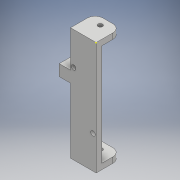
# Autodesk Inventor part: mtv_axelHolder(pushingAxel)1-13
Saved by Autodesk Inventor 2018 (Build 220112000, 112)
## iProperties
Created: 2019-01-14
Part Number: mtv_axelHolder(pushingAxel)1-13
Material: Generic
Document SubType Name: Modeling
Designer: aditya
Density: 1 g/cm^3
Appearance: Default
Author: aditya
## iProperties of the stored document mtv_axelHolder(pushingAxel)1-13_3DPrint.ipt
Created: 2019-01-14
Part Number: mtv_axelHolder(pushingAxel)1-13_3DPrint
Material: Generic
Document SubType Name: Modeling
Designer: aditya
Density: 1 g/cm^3
Appearance: Default
Author: aditya
Autodesk Inventor part; units mm, degrees
ref_plane "YZ Plane" through (0, 0, 0) normal (1, 0, 0) x (0, 1, 0)
ref_plane "XZ Plane" through (0, 0, 0) normal (0, 1, 0) x (-1, 0, 0)
ref_plane "XY Plane" through (0, 0, 0) normal (0, 0, 1) x (1, 0, 0)
sketch "Sketch1" plane through (0, 0, 0) normal (0, 1, 0) x (-1, 0, 0)
  line L0 (0, 0) -> (22.65, 0)
  line L1 (22.65, 0) -> (22.65, -100)
  line L2 (22.65, -100) -> (0, -100)
  line L3 (0, -100) -> (0, 0)
  dimension "d0" = 22.65
  dimension "d1" = 100
  constraints: 8 end point, 2 parallel, 1 horizontal, 1 perpendicular
  measures "d0" distance of L1.end L2.end
  measures "d1" distance of L0.end L1.end
extrude "Extrusion1" add sketch "Sketch1" along normal blind 5
sketch "Sketch2" plane through (0, 5, 0) normal (0, 1, 0) x (1, 0, 0)
  line L0 (-22.65, 0) -> (0, 0) projected
  line L1 (0, 0) -> (0, 100) projected
  line L2 (-22.65, 0) -> (0, 0)
  line L3 (0, 0) -> (0, 5)
  line L4 (0, 5) -> (-22.65, 5)
  line L5 (-22.65, 5) -> (-22.65, 0)
  line L6 (-22.65, 100) -> (-22.65, 0) projected
  line L7 (-22.65, 100) -> (0, 100)
  line L8 (0, 100) -> (0, 95)
  line L9 (0, 95) -> (-22.65, 95)
  line L10 (-22.65, 95) -> (-22.65, 100)
  dimension "d4" = 5
  dimension "d5" = 5
  constraints: 16 end point, 4 parallel, 2 horizontal, 2 perpendicular, 2 point on line
  measures "d4" distance of L3.end L2.end
  measures "d5" distance of L7.end L8.end
extrude "Extrusion2" add sketch "Sketch2" along normal blind 40 contours L5 L4 L1 L0 | L6 L7 L1 L9
sketch "Sketch3" plane through (-22.65, 0, 0) normal (0, 0, 1) x (1, 0, 0)
  point P0 (22.65, 0)
sketch "Sketch4" plane through (-22.65, 0, 0) normal (0, 0, 1) x (1, 0, 0)
  line L0 (22.65, 0) -> (0, 0) projected
  line L1 (22.65, 0) -> (0, 0)
  line L2 (0, 0) -> (11.325, 0)
  line L3 (11.325, 0) -> (11.325, 45)
  line L4 (22.65, 45) -> (0, 45) projected
  line L5 (0, 5) -> (22.65, 5) projected
  line L6 (22.65, 5) -> (0, 5)
  line L7 (11.325, 5) -> (11.325, 15) construction
  dimension "d8" = 10
  constraints: 10 end point, 3 midpoint, 1 collinear, 1 horizontal, 1 point on line
  measures "d8" distance of L7.start L7.end
hole "Hole1" at (-11.325, 15, 0) direction (0, 0, -1) diameter 4 depth 115 tip angle 118
sketch "Sketch5" plane through (-22.65, 0, 0) normal (0, 0, 1) x (1, 0, 0)
  line L0 (0, 5) -> (0, 45) projected
  line L1 (0, 45) -> (23, 45)
  line L2 (23, 45) -> (23, 21.7538)
  line L3 (23, 21.7538) -> (0, 21.7538)
  line L4 (0, 21.7538) -> (0, 45)
  point P0 (22.65, 0)
  dimension "d16" = 23
  constraints: 8 end point, 2 parallel, 1 horizontal, 1 perpendicular
  measures "d16" distance of L2.end L3.end
extrude "Extrusion3" cut sketch "Sketch5" against normal blind 102.75
sketch "Sketch6" plane through (0, 5, 0) normal (0, 1, 0) x (1, 0, 0)
  line L0 (0, 95) -> (-22.65, 95) construction
  line L1 (-22.65, 5) -> (0, 5) construction
  line L2 (0, 95) -> (0, 5) construction
  line L3 (0, 5) -> (-1.175, 5) construction
  line L4 (-1.175, 5) -> (-1.175, 95) construction
  line L5 (-1.175, 50) -> (-22.65, 50) construction
  line L6 (-22.65, 95) -> (-22.65, 5) construction
  line L7 (0, 5) -> (0, 95) construction
  line L8 (0, 5) -> (-22.65, 5) construction
  line L9 (-13.325, 5) -> (-9.325, 5) construction
  line L10 (-11.325, 5) -> (-11.325, 95) construction
  line L11 (-11.325, 50) -> (-2.825, 50) construction
  line L12 (-2.825, 50) -> (-2.825, 71) construction
  line L13 (-11.325, 50) -> (-19.825, 50) construction
  line L14 (-11.325, 50) -> (-2.825, 50) construction
  line L15 (-19.825, 50) -> (-19.825, 29) construction
  point P0 (0, 0)
  dimension "d19" = 1.175
  dimension "d20" = 8.5
  dimension "d21" = 21
  dimension "d22" = 90
  dimension "d23" = 8.5
  dimension "d24" = 180
  dimension "d25" = 21
  constraints: 22 end point, 5 midpoint, 3 coincident, 2 collinear, 2 parallel, 2 perpendicular, 2 point on line, 1 horizontal, 1 vertical
  measures "d19" distance of L1.end L3.end
  measures "d20" distance of L11.start L11.end
  measures "d21" distance of L11.end L12.end
  measures "d22" angle of L12 L11
  measures "d23" distance of L11.start L13.end
  measures "d24" angle of L13 L14
  measures "d25" distance of L13.end L15.end
hole "Hole2" at (-2.825, 5, -71) at (-19.825, 5, -29) direction (0, -1, 0) diameter 4 depth 115 tip angle 118
fillet "Fillet1" radius 1 2 edges at (-2.825, 5, -73) (-19.825, 5, -31)
sketch "Sketch7" plane through (0, 5, 0) normal (0, 1, 0) x (1, 0, 0)
  circle A0 centre (-2.825, 71) radius 2 construction
  line L0 (-2.825, 71) -> (-22.65, 71) construction
  line L1 (-22.65, 0) -> (-22.65, 100) construction
  circle A1 centre (-19.825, 29) radius 2 construction
  line L2 (-19.825, 29) -> (-19.825, 32.5) construction
  line L3 (-19.825, 32.5) -> (-35.65, 32.5) construction
  line L4 (-22.65, 32.5) -> (-32.65, 32.5) construction
  line L5 (-32.65, 32.5) -> (-32.65, 42.5) construction
  line L6 (-32.65, 42.5) -> (-22.65, 42.5) construction
  line L7 (-22.65, 42.5) -> (-22.65, 32.5) construction
  line L8 (-22.65, 42.5) -> (-32.65, 42.5)
  line L9 (-32.65, 42.5) -> (-32.65, 32.5)
  line L10 (-32.65, 32.5) -> (-22.65, 32.5)
  line L11 (-22.65, 32.5) -> (-22.65, 42.5)
  point P0 (0, 0)
  dimension "d34" = 3.5
  dimension "d35" = 15.825
  dimension "d36" = 10
  dimension "d37" = 10
  constraints: 22 end point, 4 horizontal, 4 parallel, 3 point on line, 2 perpendicular, 1 vertical
  measures "d34" distance of L2.start L2.end
  measures "d35" distance of L2.end L3.end
  measures "d36" distance of L5.end L6.end
  measures "d37" distance of L4.end L5.end
extrude "Extrusion4" add sketch "Sketch7" against normal blind 5
sketch "Sketch8" plane through (0, 5, 0) normal (0, 1, 0) x (1, 0, 0)
  line L0 (-32.65, 42.5) -> (-22.65, 42.5) projected
  line L1 (-22.65, 32.5) -> (-32.65, 32.5) projected
  line L2 (-32.65, 42.5) -> (-27.65, 42.5)
  line L3 (-27.65, 42.5) -> (-27.65, 32.5)
  line L4 (-27.65, 32.5) -> (-32.65, 32.5)
  line L5 (-32.65, 32.5) -> (-32.65, 42.5)
  point P0 (0, 0)
  dimension "d40" = 5
  constraints: 8 end point, 2 parallel, 1 horizontal, 1 midpoint, 1 perpendicular
  measures "d40" distance of L3.end L4.end
extrude "Extrusion5" add sketch "Sketch8" along normal blind 12.5
sketch "Sketch9" plane through (-32.65, 0, -42.5) normal (-1, 0, 0) x (0, 0, 1)
  line L0 (0, 17.5) -> (0, 0) construction
  line L1 (0, 17.5) -> (5, 17.5) construction
  line L2 (10, 17.5) -> (0, 17.5) construction
  line L3 (10, 0) -> (0, 0) construction
  line L4 (5, 0) -> (5, 17.5) construction
  point P0 (42.5, 0)
  point P1 (5, 12.5)
  constraints: 4 end point, 2 midpoint, 1 perpendicular, 1 point on line
hole "Hole3" at (-32.65, 12.5, -37.5) direction (1, 0, 0) diameter 6 depth 115 tip angle 118
fillet "Fillet2" radius 7 4 edges at (-22.65, 21.7538, -97.5) (-22.65, 21.7538, -2.5) (0, 21.7538, -2.5) (0, 21.7538, -97.5)
body "Solid1"
